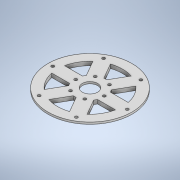
# Autodesk Inventor part: Diffuser_Filter_Holder
Saved by Autodesk Inventor 2020 (Build 240168000, 168)
## iProperties
Created: 2021-04-25
Part Number: Diffuser_Filter_Holder
Material: Generic
Document SubType Name: Modeling
Designer: Workshop
Density: 1 g/cm^3
Appearance: Default
Author: Workshop
Autodesk Inventor part; units mm, degrees
ref_plane "YZ Plane" through (0, 0, 0) normal (1, 0, 0) x (0, 1, 0)
ref_plane "XZ Plane" through (0, 0, 0) normal (0, 1, 0) x (-1, 0, 0)
ref_plane "XY Plane" through (0, 0, 0) normal (0, 0, 1) x (1, 0, 0)
sketch "Sketch1" plane through (0, 0, 0) normal (0, 0, 1) x (1, 0, 0)
  circle A0 centre (0, 0) radius 44
  circle A1 centre (0, 0) radius 34
  circle A2 centre (0, 0) radius 8
  circle A3 centre (14.925, 0) radius 1.5
  circle A4 centre (7.4625, 12.9254) radius 1.5
  circle A5 centre (-7.4625, 12.9254) radius 1.5
  circle A6 centre (-14.925, 0) radius 1.5
  circle A7 centre (-7.4625, -12.9254) radius 1.5
  circle A8 centre (7.4625, -12.9254) radius 1.5
  circle A9 centre (39, 0) radius 1.5
  line L0 (-9.2376, 16) -> (9.2376, 16)
  line L1 (9.2376, 16) -> (18.4752, 0)
  line L2 (18.4752, 0) -> (9.2376, -16)
  line L3 (9.2376, -16) -> (-9.2376, -16)
  line L4 (-9.2376, -16) -> (-18.4752, 0)
  line L5 (-18.4752, 0) -> (-9.2376, 16)
  line L6 (-1.5, 16) -> (-10.8634, 32.2178)
  line L7 (1.5, 16) -> (10.8634, 32.2178)
  line L8 (0, 0) -> (0, 44) construction
  line L9 (-13.1064, 9.299) -> (-22.4698, 25.5169)
  line L10 (-14.6064, 6.701) -> (-33.3331, 6.701)
  line L11 (-14.6064, -6.701) -> (-33.3331, -6.701)
  line L12 (-13.1064, -9.299) -> (-22.4698, -25.5169)
  line L13 (-1.5, -16) -> (-10.8634, -32.2178)
  line L14 (1.5, -16) -> (10.8634, -32.2178)
  line L15 (13.1064, -9.299) -> (22.4698, -25.5169)
  line L16 (14.6064, -6.701) -> (33.3331, -6.701)
  line L17 (14.6064, 6.701) -> (33.3331, 6.701)
  line L18 (13.1064, 9.299) -> (22.4698, 25.5169)
  circle A10 centre (19.5, 33.775) radius 1.5
  circle A11 centre (-19.5, 33.775) radius 1.5
  circle A12 centre (-39, 0) radius 1.5
  circle A13 centre (-19.5, -33.775) radius 1.5
  circle A14 centre (19.5, -33.775) radius 1.5
  dimension "d0" = 88
  dimension "d1" = 68
  dimension "d2" = 16
  dimension "d3" = 3
  dimension "d4" = 14.925
  dimension "d7" = 360
  dimension "d9" = 3
  dimension "d10" = 39
  dimension "d11" = 32
  dimension "d12" = 3
  dimension "d13" = 1.5
  dimension "d14" = 30
  dimension "d15" = 30
  dimension "d18" = 360
  dimension "d22" = 360
  constraints: 38 end point, 14 centre point, 4 coincident, 3 horizontal alignment, 2 point on circle, 2 point on line, 1 vertical, 1 vertical alignment, 78 other
  measures "d1" diameter of A1
  measures "d2" diameter of A2
  measures "d3" diameter of A3
  measures "d4" distance of A3.centre point (0, 0)
  measures "d9" diameter of A9
  measures "d10" distance of A9.centre point (0, 0)
  measures "d11" distance between parallel lines of L0 L3
  measures "d12" distance of L7.start L6.start
  measures "d13" horizontal distance of point (0, 0) L6.start
  measures "d14" angle of L8 L7
  measures "d15" angle of L6 L8
extrude "Extrusion1" add sketch "Sketch1" along normal blind 2 contours A0 | A1 L16 L2 L1 L17 | L18 L1 L0 L7 A1 | L1 L2 L3 L4 L5 L0 | A1 L14 L3 L2 L15 | L6 L0 L5 L9 A1 | A1 L12 L4 L3 L13 | L10 L5 L4 L11 A1
sketch "Sketch2" plane through (0, 0, 2) normal (0, 0, 1) x (1, 0, 0)
  circle A0 centre (0, 0) radius 44 projected
  line L0 (13.1064, 9.299) -> (22.4698, 25.5169) projected
  arc A1 (33.3331, 6.701) -> (22.4698, 25.5169) centre (0, 0) ccw projected
  line L1 (33.3331, 6.701) -> (14.6064, 6.701) projected
  line L2 (14.6064, 6.701) -> (13.1064, 9.299) projected
  line L3 (10.8634, 32.2178) -> (1.5, 16) projected
  line L4 (1.5, 16) -> (-1.5, 16) projected
  line L5 (-1.5, 16) -> (-10.8634, 32.2178) projected
  arc A2 (10.8634, 32.2178) -> (-10.8634, 32.2178) centre (0, 0) ccw projected
  arc A3 (-22.4698, 25.5169) -> (-33.3331, 6.701) centre (0, 0) ccw projected
  line L6 (-22.4698, 25.5169) -> (-13.1064, 9.299) projected
  line L7 (-13.1064, 9.299) -> (-14.6064, 6.701) projected
  line L8 (-14.6064, 6.701) -> (-33.3331, 6.701) projected
  line L9 (-14.6064, -6.701) -> (-13.1064, -9.299) projected
  line L10 (-13.1064, -9.299) -> (-22.4698, -25.5169) projected
  arc A4 (-33.3331, -6.701) -> (-22.4698, -25.5169) centre (0, 0) ccw projected
  line L11 (-33.3331, -6.701) -> (-14.6064, -6.701) projected
  line L12 (-10.8634, -32.2178) -> (-1.5, -16) projected
  line L13 (-1.5, -16) -> (1.5, -16) projected
  line L14 (1.5, -16) -> (10.8634, -32.2178) projected
  arc A5 (-10.8634, -32.2178) -> (10.8634, -32.2178) centre (0, 0) ccw projected
  circle A6 centre (0, 0) radius 8 projected
  circle A7 centre (7.4625, 12.9254) radius 1.5 projected
  circle A8 centre (14.925, 0) radius 1.5 projected
  circle A9 centre (-7.4625, 12.9254) radius 1.5 projected
  circle A10 centre (7.4625, -12.9254) radius 1.5 projected
  circle A11 centre (-14.925, 0) radius 1.5 projected
  circle A12 centre (-7.4625, -12.9254) radius 1.5 projected
  line L15 (14.6064, -6.701) -> (33.3331, -6.701) projected
  arc A13 (22.4698, -25.5169) -> (33.3331, -6.701) centre (0, 0) ccw projected
  line L16 (22.4698, -25.5169) -> (13.1064, -9.299) projected
  line L17 (13.1064, -9.299) -> (14.6064, -6.701) projected
  circle A14 centre (39, 0) radius 1.5 projected
  circle A15 centre (19.5, -33.775) radius 1.5 projected
  circle A16 centre (19.5, 33.775) radius 1.5 projected
  circle A17 centre (-19.5, 33.775) radius 1.5 projected
  circle A18 centre (-39, 0) radius 1.5 projected
  circle A19 centre (-19.5, -33.775) radius 1.5 projected
  line L18 (2.6547, 14) -> (13.7747, 33.2604)
  arc A20 (13.7747, 33.2604) -> (-13.7747, 33.2604) centre (0, 0) ccw
  line L19 (-13.7747, 33.2604) -> (-2.6547, 14)
  line L20 (-2.6547, 14) -> (2.6547, 14)
  line L21 (21.917, 28.5595) -> (10.797, 9.299)
  line L22 (10.797, 9.299) -> (13.4517, 4.701)
  line L23 (13.4517, 4.701) -> (35.6917, 4.701)
  arc A21 (35.6917, 4.701) -> (21.917, 28.5595) centre (0, 0) ccw
  line L24 (35.6917, -4.701) -> (13.4517, -4.701)
  line L25 (13.4517, -4.701) -> (10.797, -9.299)
  line L26 (10.797, -9.299) -> (21.917, -28.5595)
  arc A22 (21.917, -28.5595) -> (35.6917, -4.701) centre (0, 0) ccw
  line L27 (-21.917, -28.5595) -> (-10.797, -9.299)
  line L28 (-10.797, -9.299) -> (-13.4517, -4.701)
  line L29 (-13.4517, -4.701) -> (-35.6917, -4.701)
  arc A23 (-35.6917, -4.701) -> (-21.917, -28.5595) centre (0, 0) ccw
  arc A24 (-21.917, 28.5595) -> (-35.6917, 4.701) centre (0, 0) ccw
  line L30 (-21.917, 28.5595) -> (-10.797, 9.299)
  line L31 (-10.797, 9.299) -> (-13.4517, 4.701)
  line L32 (-13.4517, 4.701) -> (-35.6917, 4.701)
  line L33 (-2.6547, -14) -> (-13.7747, -33.2604)
  arc A25 (-13.7747, -33.2604) -> (13.7747, -33.2604) centre (0, 0) ccw
  line L34 (13.7747, -33.2604) -> (2.6547, -14)
  line L35 (2.6547, -14) -> (-2.6547, -14)
  dimension "d26" = 2
  constraints: 36 end point, 12 point on circle, 6 centre point, 5 equal length, 18 other
  measures "d26" distance between parallel lines of L3 L18
extrude "Extrusion2" add sketch "Sketch2" along normal blind 2 contours L20 L19 A20 L18 | A21 L23 L22 L21 | A22 L26 L25 L24 | A23 L29 L28 L27 | L30 L31 L32 A24 | L35 L34 A25 L33
equation "\"d13\" = 0.5 * d12"
body "Solid1"
